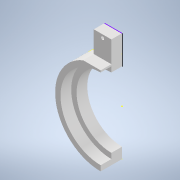
# Autodesk Inventor part: ARML
Saved by Autodesk Inventor 2020 (Build 240168000, 168)
## iProperties
Created: 2023-03-07
Part Number: ARML
Material: 一般
Document SubType Name: Modeling
Designer: robot
Density: 1 g/cm^3
Appearance: 預設
Author: robot
Autodesk Inventor part; units mm, degrees
ref_plane "YZ Plane" through (0, 0, 0) normal (1, 0, 0) x (0, 1, 0)
ref_plane "XZ Plane" through (0, 0, 0) normal (0, 1, 0) x (-1, 0, 0)
ref_plane "XY Plane" through (0, 0, 0) normal (0, 0, 1) x (1, 0, 0)
sketch "草圖1" plane through (0, 0, 0) normal (0, 0, 1) x (1, 0, 0)
  arc A0 (0, 32.5) -> (0, -32.5) centre (0, 0) ccw
  arc A1 (0, 37.5) -> (0, -37.5) centre (0, 0) ccw
  arc A2 (0, 42.5) -> (0, -42.5) centre (0, 0) ccw
  line L0 (0, 0) -> (0, -59.8463)
  line L1 (0, -59.8463) -> (0, 72.1748)
  point P0 (0, -37.5)
  point P1 (0, -42.5)
  dimension "d22" = 32.5
  dimension "d23" = 37.5
  dimension "d24" = 42.5
  constraints: 7 point on line, 6 point on circle, 4 end point, 3 centre point, 3 coincident, 1 vertical
  measures "d22" radius of A0
  measures "d23" radius of A1
  measures "d24" radius of A2
extrude "擠出1" add sketch "草圖1" against normal blind 10 contours A0 L0 A1 L1
extrude "擠出2" add sketch "草圖1" along normal mid plane 20 contours A1 L0 A2 L1
sketch "草圖2" plane through (0, 0, -10) normal (0, 0, -1) x (1, 0, 0)
  line L0 (0, -42.5) -> (0, -32.5) projected
  line L1 (0, -42.5) -> (0, -32.5)
  arc A0 (0, 42.5) -> (0, -42.5) centre (0, 0) ccw projected
  line L2 (-16.4109, -59.2037) -> (0, -59.2037)
  line L3 (0, -59.2037) -> (0, -42.5)
  line L4 (-16.4109, -39.2037) -> (-16.4109, -59.2037)
  dimension "d4" = 10
  dimension "d16" = 20
  constraints: 8 end point, 2 vertical, 1 horizontal, 1 perpendicular, 1 point on circle
  measures "d4" distance of L0.start L1.end
  measures "d16" distance of L4.start L2.start
extrude "擠出3" add sketch "草圖2" against normal blind 20
sketch "草圖4" plane through (0, 0, -10) normal (0, 0, -1) x (1, 0, 0)
  line L0 (3, 24.6083) -> (3, 21.6083)
  line L1 (0, -59.2037) -> (0, -32.5) projected
  line L2 (0, 21.6083) -> (3, 21.6083)
  circle A0 centre (3, 21.6083) radius 1.5
  line L3 (0, -59.2037) -> (-16.4109, -59.2037) projected
  line L4 (-16.4109, -59.2037) -> (-8.2055, -59.2037)
  line L5 (-8.2055, -56.2037) -> (-8.2055, -59.2037)
  line L6 (-16.4109, -59.2037) -> (-16.4109, -39.2037) projected
  circle A1 centre (-8.2055, -56.2037) radius 1.5
  point P0 (0, 0)
  point P1 (0, 24.3333)
  point P2 (0, 13.1972)
  point P3 (0, -15.5384)
  dimension "d10" = 3
  dimension "d11" = 3
  dimension "d12" = 3
  dimension "d17" = 3
  dimension "d18" = 3
  constraints: 8 end point, 2 centre point, 2 coincident, 1 midpoint, 1 parallel, 1 perpendicular, 1 point on line, 1 vertical
  measures "d10" distance of L0.start L0.end
  measures "d11" distance of L2.start L0.end
  measures "d12" diameter of A0
  measures "d17" distance of L5.start L4.end
  measures "d18" diameter of A1
extrude "擠出4" cut sketch "草圖4" against normal blind 20 contours A1
sketch "草圖6" plane through (-16.4109, 39.2037, -10) normal (-1, 0, 0) x (0, 0, 1)
  line L0 (0, 20) -> (20, 20) projected
  line L1 (20, 20) -> (10, 20)
  line L2 (10, 20) -> (10, 0)
  line L3 (20, 0) -> (0, 0) projected
  line L4 (20, 20) -> (20, 0) projected
  line L5 (10, 20) -> (20, 20)
  line L6 (20, 20) -> (20, 0)
  line L7 (20, 0) -> (10, 0)
  line L8 (10, 0) -> (10, 20)
  point P0 (10, -39.2037)
  dimension "d19" = 10
  constraints: 12 end point, 2 midpoint, 2 parallel, 1 horizontal, 1 perpendicular, 1 vertical
  measures "d19" distance of L0.end L1.end
extrude "擠出5" cut sketch "草圖6" against normal blind 20
